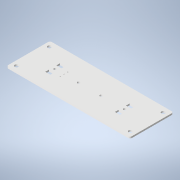
# Autodesk Inventor part: Interstage A
Saved by Autodesk Inventor 2020.3 (Build 243373000, 373)
## iProperties
Created: 2020-05-18
Part Number: Interstage A
Material: Genérico
Document SubType Name: Modeling
Designer: javic
Density: 1 g/cm^3
Appearance: Valor por defecto
Mass: 2.45575 g
Surface Area: 50.0845 cm^2
Volume: 2.45575 cm^3
Author: javic
Autodesk Inventor part; units mm, degrees
ref_plane "YZ Plane" through (0, 0, 0) normal (1, 0, 0) x (0, 1, 0)
ref_plane "XZ Plane" through (0, 0, 0) normal (0, 1, 0) x (-1, 0, 0)
ref_plane "XY Plane" through (0, 0, 0) normal (0, 0, 1) x (1, 0, 0)
sketch "Boceto1" plane through (0, 0, 0) normal (0, 1, 0) x (-1, 0, 0)
  arc A0 (-1.27, 1.27) -> (0, 0) centre (0, 1.27) ccw
  line L0 (0, 0) -> (79.96, 0)
  arc A1 (79.96, 0) -> (81.23, 1.27) centre (79.96, 1.27) ccw
  line L1 (81.23, 1.27) -> (81.23, 27.73)
  arc A2 (81.23, 27.73) -> (79.96, 29) centre (79.96, 27.73) ccw
  line L2 (79.96, 29) -> (0, 29)
  arc A3 (0, 29) -> (-1.27, 27.73) centre (0, 27.73) ccw
  line L3 (-1.27, 27.73) -> (-1.27, 1.27)
  circle A4 centre (77.98, 3.5) radius 1.25
  circle A5 centre (1.98, 25.5) radius 1.25
  circle A6 centre (1.98, 3.5) radius 1.25
  circle A7 centre (77.98, 25.5) radius 1.25
  circle A8 centre (47.48, 14.5) radius 0.9
  circle A9 centre (32.48, 14.5) radius 0.9
  point P0 (0, 0)
  constraints: 10 centre point, 8 end point, 8 point on circle, 8 tangent, 7 equal radius, 2 perpendicular, 1 parallel
extrude "Extrusión1" add sketch "Boceto1" along normal blind 1.04
sketch "Boceto3" plane through (0, 1.04, 0) normal (0, 1, 0) x (1, 0, 0)
  circle A0 centre (-63.23, -14.5) radius 0.9
  circle A1 centre (-16.73, -14.5) radius 0.9
  line L0 (-81.23, -1.27) -> (-81.23, -27.73) projected
  line L1 (0, 0) -> (-79.96, 0) projected
  line L2 (1.27, -27.73) -> (1.27, -1.27) projected
  line L3 (-79.96, -29) -> (0, -29) projected
  dimension "d15" = 1.8
  dimension "d16" = 1.8
  dimension "d17" = 18
  dimension "d18" = 14.5
  dimension "d19" = 18
  dimension "d20" = 14.5
  constraints: 2 centre point
  measures "d15" diameter of A0
  measures "d16" diameter of A1
  measures "d17" distance from line of L0 A0.centre
  measures "d18" distance from line of L1 A0.centre
  measures "d19" distance from line of L2 A1.centre
  measures "d20" distance from line of L3 A1.centre
hole "Agujero2" at (-63.23, 1.04, 14.5) at (-16.73, 1.04, 14.5) direction (0, -1, 0) diameter 1.8 end through all
sketch "Boceto4" plane through (0, 1.04, 0) normal (0, 1, 0) x (1, 0, 0)
  circle A0 centre (-57.13, -17.04) radius 0.4
  line L0 (-81.23, -1.27) -> (-81.23, -27.73) projected
  line L1 (-79.96, -29) -> (0, -29) projected
  circle A1 centre (-57.13, -14.5) radius 0.4
  circle A2 centre (-57.13, -11.96) radius 0.4
  line L2 (0, 0) -> (-79.96, 0) projected
  dimension "d28" = 0.8
  dimension "d29" = 24.1
  dimension "d30" = 11.96
  dimension "d31" = 0.8
  dimension "d32" = 0.8
  dimension "d33" = 11.96
  dimension "d34" = 2.54
  dimension "d35" = 2.54
  constraints: 3 centre point
  measures "d28" diameter of A0
  measures "d29" distance from line of L0 A0.centre
  measures "d30" distance from line of L1 A0.centre
  measures "d31" diameter of A1
  measures "d32" diameter of A2
  measures "d33" distance from line of L2 A2.centre
  measures "d34" distance of A1.centre A0.centre
  measures "d35" distance of A2.centre A1.centre
hole "Agujero3" at (-57.13, 1.04, 17.04) at (-57.13, 1.04, 14.5) at (-57.13, 1.04, 11.96) direction (0, -1, 0) diameter 0.8 end through all
sketch "Boceto5" plane through (0, 0, 0) normal (0, -1, 0) x (1, 0, 0)
  line L0 (-15.03, 9.6) -> (-18.43, 9.6)
  line L1 (-18.43, 9.6) -> (-18.43, 12)
  line L2 (-18.43, 12) -> (-15.03, 12)
  line L3 (-15.03, 12) -> (-15.03, 9.6)
  line L4 (-79.96, 29) -> (0, 29) projected
  line L5 (1.27, 27.73) -> (1.27, 1.27) projected
  line L6 (-15.03, 17) -> (-18.43, 17)
  line L7 (-18.43, 17) -> (-18.43, 19.4)
  line L8 (-18.43, 19.4) -> (-15.03, 19.4)
  line L9 (-15.03, 19.4) -> (-15.03, 17)
  line L10 (0, 0) -> (-79.96, 0) projected
  line L11 (-61.53, 9.6) -> (-64.93, 9.6)
  line L12 (-64.93, 9.6) -> (-64.93, 12)
  line L13 (-64.93, 12) -> (-61.53, 12)
  line L14 (-61.53, 12) -> (-61.53, 9.6)
  line L15 (-81.23, 1.27) -> (-81.23, 27.73) projected
  line L16 (-61.53, 17) -> (-64.93, 17)
  line L17 (-64.93, 17) -> (-64.93, 19.4)
  line L18 (-64.93, 19.4) -> (-61.53, 19.4)
  line L19 (-61.53, 19.4) -> (-61.53, 17)
  dimension "d43" = 3.4
  dimension "d44" = 2.4
  dimension "d47" = 16.3
  dimension "d48" = 2.4
  dimension "d49" = 9.6
  dimension "d50" = 9.6
  dimension "d51" = 3.4
  dimension "d52" = 2.4
  dimension "d53" = 9.6
  dimension "d54" = 16.3
  dimension "d55" = 3.4
  dimension "d56" = 2.4
  dimension "d57" = 16.3
  dimension "d58" = 9.6
  constraints: 32 end point, 8 parallel, 4 horizontal, 4 perpendicular
  measures "d43" distance of L1.end L2.end
  measures "d44" distance of L0.end L1.end
  measures "d47" distance between parallel lines of L5 L3
  measures "d48" distance of L6.end L7.end
  measures "d49" distance between parallel lines of L4 L8
  measures "d50" distance between parallel lines of L10 L0
  measures "d51" distance of L12.end L13.end
  measures "d52" distance of L11.end L12.end
  measures "d53" distance between parallel lines of L11 L10
  measures "d54" distance between parallel lines of L15 L12
  measures "d55" distance of L17.end L18.end
  measures "d56" distance of L16.end L17.end
  measures "d57" distance between parallel lines of L15 L17
  measures "d58" distance between parallel lines of L4 L18
extrude "Extrusión2" cut sketch "Boceto5" against normal through all
sketch "Boceto6" plane through (0, 0, 0) normal (0, -1, 0) x (1, 0, 0)
  point P0 (0, 0)
